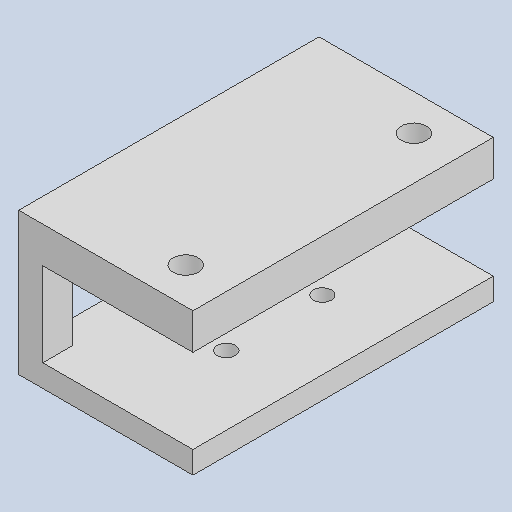
# Autodesk Inventor part: креп_центр_ролик
Saved by Autodesk Inventor 2023.1 (Build 271208000, 208)
## iProperties
Created: 2025-12-22
Part Number: креп_центр_ролик
Material: Типовые
Document SubType Name: Modeling
Designer: DELL
Density: 1 g/cm^3
Appearance: По умолчанию
Author: DELL
Autodesk Inventor part; units mm, degrees
ref_plane "YZ Plane" through (0, 0, 0) normal (1, 0, 0) x (0, 1, 0)
ref_plane "XZ Plane" through (0, 0, 0) normal (0, 1, 0) x (-1, 0, 0)
ref_plane "XY Plane" through (0, 0, 0) normal (0, 0, 1) x (1, 0, 0)
sketch "Эскиз1" plane through (0, 0, 0) normal (0, 0, 1) x (1, 0, 0)
  line L0 (12.5, 7) -> (-12.5, 7)
  line L1 (-12.5, 7) -> (-12.5, -7)
  line L2 (-12.5, -7) -> (12.5, -7)
  line L3 (12.5, -7) -> (12.5, 7)
  line L4 (12.5, 7) -> (-12.5, -7) construction
  line L5 (-12.5, 7) -> (12.5, -7) construction
  line L6 (-16.5, 13) -> (12.5, 13)
  line L7 (11.5, 13) -> (11.5, -10.7) construction
  line L8 (11.5, -10.7) -> (12.5, -10.7) construction
  line L9 (-16.5, -10.7) -> (-16.5, 13)
  line L10 (12.5, -7) -> (12.5, -10.7)
  line L11 (12.5, 7) -> (12.5, 13)
  line L12 (12.5, 13) -> (11.5, 13) construction
  line L13 (12.5, -10.7) -> (-16.5, -10.7)
  point P0 (0, 0)
  dimension "d0" = 25
  dimension "d1" = 14
  dimension "d2" = 6
  dimension "d11" = 3.7
  constraints: 28 end point, 7 parallel, 5 perpendicular, 2 midpoint, 1 horizontal, 1 point on line
  measures "d0" distance of L2.end L1.end
  measures "d1" distance of L1.end L0.end
  measures "d2" distance between parallel lines of L0 L6
  measures "d11" distance between parallel lines of L13 L2
extrude "Выдавливание1" add sketch "Эскиз1" along normal blind 50 contours L0 L1 L2 L10 L13 L9 L6 L11
sketch "Эскиз2" plane through (-16.5, -10.7, 0) normal (-1, 0, 0) x (0, 0, 1)
  line L0 (0, 23.7) -> (0, 0) construction
  line L1 (0, 0) -> (50, 0) construction
  line L2 (50, 23.7) -> (50, 0) construction
  line L3 (0, 23.7) -> (50, 23.7) construction
  line L4 (45, 19.7) -> (5, 19.7)
  line L5 (5, 19.7) -> (5, 4)
  line L6 (45, 4) -> (45, 19.7)
  line L7 (45, 19.7) -> (5, 4) construction
  line L8 (5, 19.7) -> (45, 4) construction
  line L9 (0, 23.7) -> (50, 23.7) projected
  line L10 (50, 0) -> (50, 3.7) projected
  line L11 (0, 23.7) -> (50, 0) construction
  line L12 (5, 3.7) -> (45, 3.7)
  line L13 (5, 4) -> (5, 3.7)
  line L14 (0, 3.7) -> (50, 3.7) projected
  line L15 (45, 4) -> (45, 3.7)
  point P0 (0, 10.7)
  point P1 (25, 11.85)
  dimension "d5" = 40
  dimension "d6" = 4
  dimension "d12" = 3.7
  constraints: 18 end point, 3 midpoint, 3 perpendicular, 2 horizontal, 1 parallel
  measures "d5" distance of L6.start L5.end
  measures "d6" distance between parallel lines of L3 L4
  measures "d12" distance between parallel lines of L12 L1
extrude "Выдавливание2" cut sketch "Эскиз2" against normal blind 4
sketch "Эскиз4" plane through (-16.5, -10.7, 0) normal (0, -1, 0) x (1, 0, 0)
  line L0 (302.9, 12.95) -> (302.9, 38.45) construction
  line L1 (302.9, 38.45) -> (-1.5, 38.45) construction
  line L2 (-1.5, 38.45) -> (-1.5, 12.95) construction
  line L3 (-1.5, 12.95) -> (302.9, 12.95) construction
  circle A0 centre (17.5, 32.95) radius 1.5 projected
  circle A1 centre (2.5, 32.95) radius 1.5 projected
  circle A2 centre (2.5, 16.95) radius 1.5 projected
  circle A3 centre (17.5, 16.95) radius 1.5 projected
  circle A4 centre (283.9, 32.95) radius 1.5 construction
  circle A5 centre (298.9, 32.95) radius 1.5 construction
  circle A6 centre (298.9, 16.95) radius 1.5 construction
  circle A7 centre (283.9, 16.95) radius 1.5 construction
  point P0 (16.5, 0)
extrude "Выдавливание3" cut sketch "Эскиз4" against normal blind 4
sketch "Эскиз6" plane through (-16.5, 13, 0) normal (0, 1, 0) x (1, 0, 0)
  circle A0 centre (9.8, -9.6796) radius 6 construction
  line L0 (15.8, -9.6796) -> (15.8, -27.7296) construction
  circle A1 centre (21.8, -6) radius 6 construction
  circle A2 centre (21.8, -6) radius 2.1
  line L1 (29, -25) -> (0, -25) construction
  circle A3 centre (21.8, -44) radius 2.1
  dimension "d13" = 12
  dimension "d14" = 12
  dimension "d15" = 4.2
  constraints: 4 end point, 3 centre point, 2 coincident, 1 horizontal alignment, 1 symmetric about line, 1 tangent, 1 vertical, 3 other
  measures "d14" diameter of A1
  measures "d15" diameter of A2
extrude "Выдавливание4" cut sketch "Эскиз6" against normal blind 5
